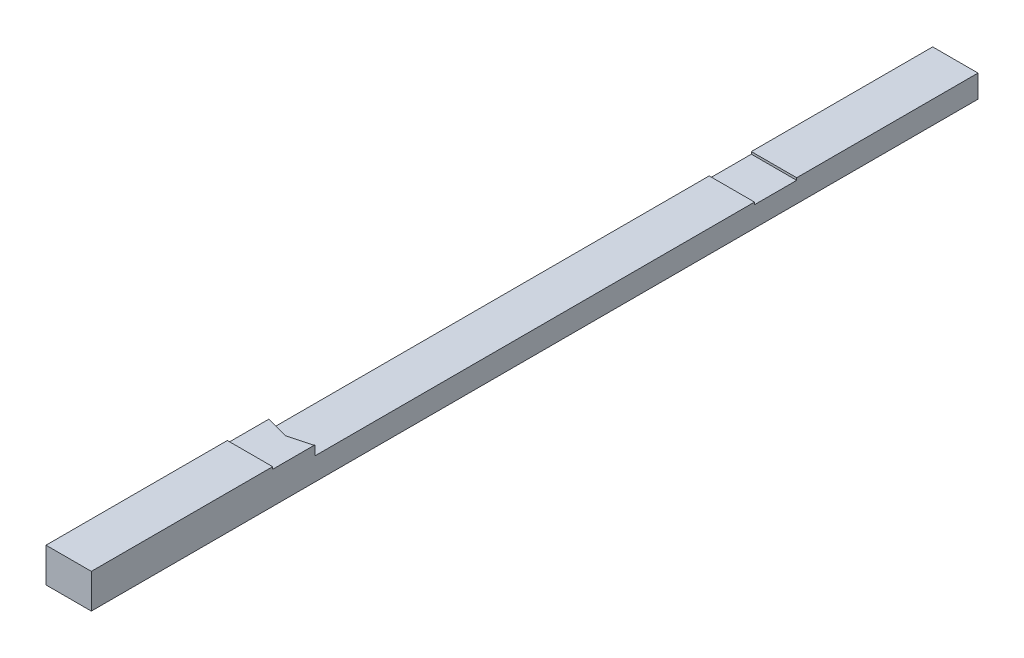
# Autodesk Inventor part: ground_all
Saved by Autodesk Inventor 2025.2 (Build 292293000, 293)
## iProperties
Created: 2025-01-19
Part Number: ground_all
Material: Типовые
Document SubType Name: Modeling
Designer: Admin
Density: 1 g/cm^3
Appearance: По умолчанию
Author: Admin
Autodesk Inventor part; units mm, degrees
ref_plane "YZ Plane" through (0, 0, 0) normal (1, 0, 0) x (0, 1, 0)
ref_plane "XZ Plane" through (0, 0, 0) normal (0, 1, 0) x (-1, 0, 0)
ref_plane "XY Plane" through (0, 0, 0) normal (0, 0, 1) x (1, 0, 0)
sketch "Эскиз1" plane through (0, 0, 0) normal (1, 0, 0) x (0, 1, 0)
  line L0 (0, 0) -> (0, -970)
  line L1 (0, -970) -> (-5, -970)
  line L2 (-5, -970) -> (-5, -1063)
  line L3 (-5, -1063) -> (0, -1063)
  line L4 (0, -1063) -> (0, -1463)
  line L5 (0, -1463) -> (-50, -1463)
  line L6 (-50, -1463) -> (-50, 493)
  line L7 (0, 0) -> (21, 0)
  line L8 (21, 0) -> (21, 93)
  line L9 (21, 93) -> (26, 93)
  line L10 (26, 93) -> (26, 493)
  line L11 (26, 493) -> (-50, 493)
  dimension "d0" = 970
  dimension "d1" = 5
  dimension "d2" = 93
  dimension "d3" = 400
  dimension "d4" = 50
  dimension "d5" = 21
  dimension "d6" = 93
  dimension "d7" = 5
  dimension "d8" = 400
  dimension "d9" = 1956
  constraints: 24 end point, 7 perpendicular, 3 vertical, 2 horizontal
  measures "d0" distance of L0.start L0.end
  measures "d1" distance of L0.end L1.end
  measures "d2" distance of L1.end L2.end
  measures "d3" distance of L3.end L4.end
  measures "d4" distance of L4.end L5.end
  measures "d5" distance of L0.start L7.end
  measures "d6" distance of L7.end L8.end
  measures "d7" distance of L8.end L9.end
  measures "d8" distance of L9.end L10.end
  measures "d9" distance of L5.end L6.end
extrude "Выдавливание1" add sketch "Эскиз1" along normal blind 100
sketch "Эскиз2" plane through (0, 21, 93) normal (0, 1, 0) x (1, 0, 0)
  line L0 (0, 91.3764) -> (49.9516, 78.389)
  line L1 (0, 93) -> (0, 91.3764)
  line L2 (0, 93) -> (99.9032, 93)
  line L3 (99.9032, 91.3764) -> (99.9032, 93)
  line L4 (49.9516, 78.389) -> (99.9032, 91.3764)
  constraints: 10 end point, 2 point on line
extrude "Выдавливание2" cut sketch "Эскиз2" against normal up to surface (21 mm away)
